Autodesk Fusion 360 part; units mm, degrees
note: some values were not read from the file. Chosen so that the rebuilt part matches the saved one: a direction; which face or edge a step refers to. Set by a fixed rule: which sketch regions a step uses; the direction of a hole.
(part 2 of 2)
component "FrontUnit" placed x (1, 0, 0) y (0, 1, 0) z (0, 0, 1) at (0, 0, 0)
component "SideUnit" placed x (1, 0, 0) y (0, 1, 0) z (0, 0, 1) at (0, 0, 0)
component "BackUnit" placed x (1, 0, 0) y (0, 1, 0) z (0, 0, 1) at (0, 0, 0)
component "BackUnitCover" placed x (1, 0, 0) y (0, 1, 0) z (0, 0, 1) at (0, 0, 0)
component "Lens(ミラー)" placed x (0, 1, 0) y (1, 0, 0) z (0, 0, -1) at (-51.8703, 21, -24.5)
component "HalfMirror(ミラー)" placed x (0, -1, 0) y (-0.707107, 0, 0.707107) z (-0.707107, 0, -0.707107) at (-49.598, 40, -44.0122)
component "Display(ミラー)" placed x (0, 1, 0) y (1, 0, 0) z (0, 0, -1) at (-103, 7.825, -33.795)
component "SideUnit(ミラー)" placed x (-1, 0, 0) y (0, 1, 0) z (0, 0, -1) at (0, 0, 0)
component "NosePart" placed x (1, 0, 0) y (0, 1, 0) z (0, 0, 1) at (0, 0, 0)
component "BoardPillar" placed x (1, 0, 0) y (0, 0, 1) z (0, -1, 0) at (-29, 36, 211)
component "BoardPillar" placed x (1, 0, 0) y (0, 0, 1) z (0, -1, 0) at (29, 36, 211)
component "BoardPillar" placed x (1, 0, 0) y (0, 0, 1) z (0, -1, 0) at (-29, 13, 211)
component "BoardPillar" placed x (1, 0, 0) y (0, 0, 1) z (0, -1, 0) at (29, 13, 211)
equation "d20 = ( 36.75 / 2 ) * 1 mm"
equation "d200 = ( 5.7 / 2 ) * 1 mm"
equation "d201 = ( 5.7 / 2 ) * 1 mm"
